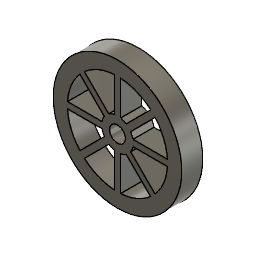
Pata (Autodesk Fusion 360 archive; units mm, degrees)
design "opción 2 rueds temporal"
Autodesk Fusion 360 part; units mm, degrees
sketch "Boceto1" plane through (0, 0, 0) normal (0, 0, 1) x (1, 0, 0)
  circle A0 centre (0, 0) radius 61
  line L0 (-47.4052, 3) -> (-14.6969, 3)
  line L1 (0, 0) -> (-2.1213, 2.1213)
  line L2 (12.5136, -8.271) -> (35.6418, -31.3992)
  line L3 (-31.3992, 35.6418) -> (-8.271, 12.5136)
  line L4 (-3, 14.6969) -> (-3, 47.4052)
  line L5 (-35.6418, 31.3992) -> (-12.5136, 8.271)
  line L6 (-14.6969, -3) -> (-47.4052, -3)
  line L7 (-35.6418, -31.3992) -> (-12.5136, -8.271)
  line L8 (-3, -47.4052) -> (-3, -14.6969)
  line L9 (-8.271, -12.5136) -> (-31.3992, -35.6418)
  line L10 (8.271, -12.5136) -> (31.3992, -35.6418)
  line L11 (3, -14.6969) -> (3, -47.4052)
  line L12 (3, 47.4052) -> (3, 14.6969)
  line L13 (47.4052, -3) -> (14.6969, -3)
  line L14 (35.6418, 31.3992) -> (12.5136, 8.271)
  line L15 (14.6969, 3) -> (47.4052, 3)
  line L16 (3, 0) -> (4.2426, 0) construction
  arc A1 (3, -14.6969) -> (8.271, -12.5136) centre (0, 0) ccw
  arc A2 (-14.6969, -3) -> (-12.5136, -8.271) centre (0, 0) ccw
  arc A3 (-8.271, -12.5136) -> (-3, -14.6969) centre (0, 0) ccw
  arc A4 (-12.5136, 8.271) -> (-14.6969, 3) centre (0, 0) ccw
  arc A5 (-3, 14.6969) -> (-8.271, 12.5136) centre (0, 0) ccw
  line L17 (31.3992, 35.6418) -> (8.271, 12.5136)
  arc A6 (12.5136, -8.271) -> (12.5136, 8.271) centre (0, 0) ccw
  arc A7 (8.271, 12.5136) -> (3, 14.6969) centre (0, 0) ccw
  arc A8 (47.4052, 3) -> (35.6418, 31.3992) centre (0, 0) ccw
  arc A9 (35.6418, -31.3992) -> (47.4052, -3) centre (0, 0) ccw
  arc A10 (3, -47.4052) -> (31.3992, -35.6418) centre (0, 0) ccw
  arc A11 (-31.3992, -35.6418) -> (-3, -47.4052) centre (0, 0) ccw
  arc A12 (-35.6418, 31.3992) -> (-47.4052, 3) centre (0, 0) ccw
  arc A13 (-47.4052, -3) -> (-35.6418, -31.3992) centre (0, 0) ccw
  arc A14 (31.3992, 35.6418) -> (3, 47.4052) centre (0, 0) ccw
  arc A15 (-3, 47.4052) -> (-31.3992, 35.6418) centre (0, 0) ccw
  circle A16 centre (0, 0) radius 7.5
  dimension "d1" = 122
  dimension "d2" = 95
  dimension "d3" = 30
  dimension "d12" = 15
  constraint coincident A0.centre L1.start
  constraint vertical L12
  constraint vertical L8
  constraint horizontal L0
  constraint horizontal L13
  constraint horizontal L16
  constraint perpendicular L1 L7
  constraint coincident L2.end A12
  constraint perpendicular L3 L14
  constraint collinear L2 L3
  constraint coincident L3.end A2
  constraint coincident L4.start A2
  constraint coincident L5.end A2
  constraint collinear L6 L13
  constraint coincident L9.start A2
  constraint collinear L9 L14
  constraint coincident L11.start A2
  constraint collinear L11 L12
  constraint coincident L17.start A12
  constraint coincident L12.end A2
  constraint coincident L14.end A2
  constraint coincident L15.start A2
  constraint coincident L13.end A2
  constraint coincident L2.start A2
  constraint concentric A2 A6
  constraint concentric A1 A2
  constraint concentric A2 A3
  constraint concentric A4 A6
  constraint concentric A5 A6
  constraint coincident L17.end A6
  constraint concentric A6 A7
  constraint concentric A12 A14
  constraint coincident L15.end A12
  constraint concentric A8 A12
  constraint concentric A9 A12
  constraint concentric A10 A12
  constraint coincident L9.end A12
  constraint concentric A11 A12
  constraint concentric A12 A13
  constraint coincident L4.end A14
  constraint concentric A14 A15
  constraint concentric A14 A16
  measures "d1" diameter of A0
  measures "d2" diameter of A12
  measures "d3" diameter of A2
  measures "d12" diameter of A16
extrude "Extruir1" add sketch "Boceto1" along normal blind 20
scale "Escala1" factor 0.82 about (-61, 0, 20) bodies 1
